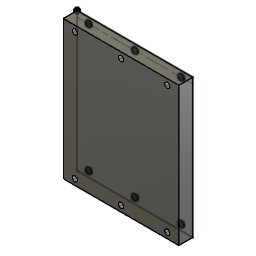
CNC_frame_mount_plate (Autodesk Fusion 360 design; units mm, degrees)
Autodesk Fusion 360 part; units mm, degrees
note: some values were not read from the file. Set by a fixed rule: which sketch regions a step uses.
sketch "Sketch1" plane through (0, 0, 0) normal (0, 0, 1) x (1, 0, 0)
  line L0 (30, 30) -> (-30, 30)
  line L1 (-30, 30) -> (-30, -30)
  line L2 (-30, -30) -> (30, -30)
  line L3 (30, -30) -> (30, 30)
  line L4 (30, 30) -> (-30, -30) construction
  line L5 (-30, 30) -> (30, -30) construction
  circle A0 centre (-30, 30) radius 2.8
  circle A1 centre (30, 30) radius 2.8
  circle A2 centre (-30, -30) radius 2.8
  circle A3 centre (30, -30) radius 2.8
  line L6 (50, 50) -> (-50, 50)
  line L7 (-50, 50) -> (-50, -50)
  line L8 (-50, -50) -> (50, -50)
  line L9 (50, -50) -> (50, 50)
  line L10 (50, 50) -> (-50, -50) construction
  line L11 (-50, 50) -> (50, -50) construction
  line L12 (50, 50) -> (-50, 50)
  line L13 (-50, 50) -> (-50, 60)
  line L14 (-50, 60) -> (50, 60)
  line L15 (50, 60) -> (50, 50)
  line L16 (50, -50) -> (-50, -50)
  line L17 (-50, -50) -> (-50, -60)
  line L18 (-50, -60) -> (50, -60)
  line L19 (50, -60) -> (50, -50)
  circle A4 centre (-30, 30) radius 2
  circle A5 centre (30, 30) radius 2
  circle A6 centre (-30, -30) radius 2
  circle A7 centre (30, -30) radius 2
  dimension "d1" = 60
  dimension "d2" = 60
  dimension "d3" = 5.6
  dimension "d6" = 60
  dimension "d7" = -60
  dimension "d8" = 100
  dimension "d9" = 100
  dimension "d12" = 100
  dimension "d13" = 10
  dimension "d14" = 100
  dimension "d15" = 10
  dimension "d26" = 4
  constraint horizontal L0
  constraint perpendicular L0 L1
  constraint parallel L0 L2
  constraint parallel L1 L3
  constraint coincident L4 origin
  constraint coincident L5 origin
  constraint coincident L0.end L1.start
  constraint horizontal L6
  constraint perpendicular L6 L7
  constraint parallel L6 L8
  constraint parallel L7 L9
  constraint coincident L10 origin
  constraint coincident L11 origin
  constraint horizontal L12
  constraint vertical L13
  constraint horizontal L14
  constraint vertical L15
  constraint horizontal L16
  constraint vertical L17
  constraint horizontal L18
  constraint vertical L19
  constraint concentric A0 A4
  measures "d1" distance of L1.end L2.end
  measures "d2" distance of L0.end L1.end
  measures "d3" diameter of A0
  measures "d8" distance of L7.end L8.end
  measures "d9" distance of L6.end L7.end
  measures "d12" distance of L6.start L6.end
  measures "d13" distance of L6.start L14.end
  measures "d14" distance of L8.end L7.end
  measures "d15" distance of L8.end L18.end
  measures "d26" diameter of A4
extrude "Extrude1" add sketch "Sketch1" along normal blind 10 contours L0 L1 L2 L3 A0 A1 A2 A3 | L6 L7 L8 L9 L12 L16 makes body 1
extrude "Extrude2" add sketch "Sketch1" along normal blind 110 contours L6 L12 L13 L14 L15 | L8 L16 L17 L18 L19 bodies 1
sketch "Sketch2" plane through (0, 0, 110) normal (0, 0, 1) x (1, 0, 0)
  line L0 (50, 60) -> (-50, 60)
  line L1 (-50, 60) -> (-50, 50)
  line L2 (-50, 50) -> (50, 50)
  line L3 (50, 50) -> (50, 60)
  circle A0 centre (-40, 55) radius 2.8
  line L4 (-50, 55) -> (50, 55)
  circle A1 centre (0, 55) radius 2.8
  circle A2 centre (40, 55) radius 2.8
  circle A3 centre (-40, -55) radius 2.8
  circle A4 centre (0, -55) radius 2.8
  circle A5 centre (40, -55) radius 2.8
  line L5 (-50, 60) -> (50, 60)
  line L6 (50, 60) -> (50, -60)
  line L7 (50, -60) -> (-50, -60)
  line L8 (-50, -60) -> (-50, 60)
  circle A6 centre (-40, 55) radius 2.25
  circle A7 centre (0, 55) radius 2.25
  circle A8 centre (40, 55) radius 2.25
  circle A9 centre (-40, -55) radius 2.25
  circle A10 centre (0, -55) radius 2.25
  circle A11 centre (40, -55) radius 2.25
  dimension "d18" = 5.6
  dimension "d19" = 10
  dimension "d22" = 40
  dimension "d23" = -110
  dimension "d30" = 120
  dimension "d31" = 100
  dimension "d32" = 4.5
  constraint midpoint L1 L4.start
  constraint midpoint L3 L4.end
  constraint coincident A0.centre L4
  constraint horizontal L5
  constraint vertical L6
  constraint horizontal L7
  constraint vertical L8
  constraint coincident L0.end L1.start
  constraint concentric A0 A6
  measures "d18" diameter of A0
  measures "d19" distance of L1 A0.centre
  measures "d30" distance of L0.end L7.end
  measures "d31" distance of L0.end L0.start
  measures "d32" diameter of A6
extrude "Extrude3" cut sketch "Sketch2" against normal blind 8.1 contours L4 A2 A8 | L4 A2 A8 | A0 L4 A6 | A0 L4 A6 | L4 A8 | L4 A8 | L4 A6 | L4 A6 | L4 A1 A7 | L4 A1 A7 | L4 A7 | L4 A7 | A3 | A4 | A5 | A9 | A10 | A11 bodies 1
extrude "Extrude4" add sketch "Sketch1" against normal blind 1.9 from surface at 10 contours L0 L1 A0 A4 | L0 L1 A0 A4 | L0 L3 A1 A5 | L0 L3 A1 A5 | L1 L2 A2 A6 | L1 L2 A2 A6 | L2 L3 A3 A7 | L2 L3 A3 A7 bodies 1
extrude "Extrude5" add sketch "Sketch2" along normal blind 12 separate body contours L0 L1 L3 A0 L4 A1 A2 L5 L6 L8 | L1 L2 L3 A0 L4 A1 A2 L6 L8 | L2 L6 L7 L8 | L4 A2 A8 | L4 A2 A8 | A0 L4 A6 | A0 L4 A6 | L4 A1 A7 | L4 A1 A7 | A3 | A4 | A5 makes body 2
chamfer "Chamfer1" distance 5 angle 45 4 edges at (-50, 0, 0) (0, 60, 0) (50, 0, 0) (0, -60, 0) on bodies 1
hidden bodies 1
